Autodesk Inventor part; units mm, degrees
(part 2 of 5)
  line L380 (98.7844, -25.841) -> (96.8773, -27.7481)
  line L381 (94.3702, -25.841) -> (96.2773, -27.7481)
  line L382 (96.5773, -27.7481) -> (96.8773, -27.7481)
  line L383 (96.5773, -27.7481) -> (96.2773, -27.7481)
  line L384 (94.0773, -25.1339) -> (94.0773, -8.3624)
  line L385 (99.0773, -8.3624) -> (99.0773, -25.1339)
  arc A154 (94.3702, -7.6553) -> (94.0773, -8.3624) centre (95.0773, -8.3624) ccw
  line L386 (94.3702, -7.6553) -> (96.2773, -5.7481)
  line L387 (96.5773, -5.7481) -> (96.2773, -5.7481)
  line L388 (96.5773, -5.7481) -> (96.8773, -5.7481)
  arc A155 (99.0773, -8.3624) -> (98.7844, -7.6553) centre (98.0773, -8.3624) ccw
  line L389 (98.7844, -7.6553) -> (96.8773, -5.7481)
  arc A156 (123.5844, -1.041) -> (123.8773, -0.3339) centre (122.8773, -0.3339) ccw
  arc A157 (118.8773, -0.3339) -> (119.1702, -1.041) centre (119.8773, -0.3339) ccw
  line L390 (123.5844, -1.041) -> (121.6773, -2.9481)
  line L391 (119.1702, -1.041) -> (121.0773, -2.9481)
  line L392 (121.3773, -2.9481) -> (121.6773, -2.9481)
  line L393 (121.3773, -2.9481) -> (121.0773, -2.9481)
  line L394 (118.8773, -0.3339) -> (118.8773, 16.4376)
  line L395 (123.8773, 16.4376) -> (123.8773, -0.3339)
  arc A158 (119.1702, 17.1447) -> (118.8773, 16.4376) centre (119.8773, 16.4376) ccw
  line L396 (119.1702, 17.1447) -> (121.0773, 19.0519)
  line L397 (121.3773, 19.0519) -> (121.0773, 19.0519)
  line L398 (121.3773, 19.0519) -> (121.6773, 19.0519)
  arc A159 (123.8773, 16.4376) -> (123.5844, 17.1447) centre (122.8773, 16.4376) ccw
  line L399 (123.5844, 17.1447) -> (121.6773, 19.0519)
  arc A160 (123.5844, -25.841) -> (123.8773, -25.1339) centre (122.8773, -25.1339) ccw
  arc A161 (118.8773, -25.1339) -> (119.1702, -25.841) centre (119.8773, -25.1339) ccw
  line L400 (123.5844, -25.841) -> (121.6773, -27.7481)
  line L401 (119.1702, -25.841) -> (121.0773, -27.7481)
  line L402 (121.3773, -27.7481) -> (121.6773, -27.7481)
  line L403 (121.3773, -27.7481) -> (121.0773, -27.7481)
  line L404 (118.8773, -25.1339) -> (118.8773, -8.3624)
  line L405 (123.8773, -8.3624) -> (123.8773, -25.1339)
  arc A162 (119.1702, -7.6553) -> (118.8773, -8.3624) centre (119.8773, -8.3624) ccw
  line L406 (119.1702, -7.6553) -> (121.0773, -5.7481)
  line L407 (121.3773, -5.7481) -> (121.0773, -5.7481)
  line L408 (121.3773, -5.7481) -> (121.6773, -5.7481)
  arc A163 (123.8773, -8.3624) -> (123.5844, -7.6553) centre (122.8773, -8.3624) ccw
  line L409 (123.5844, -7.6553) -> (121.6773, -5.7481)
  arc A164 (99.8844, -31.3553) -> (100.5916, -31.6481) centre (100.5916, -30.6481) ccw
  arc A165 (100.5916, -26.6481) -> (99.8844, -26.941) centre (100.5916, -27.6481) ccw
  line L410 (99.8844, -31.3553) -> (97.9773, -29.4481)
  line L411 (99.8844, -26.941) -> (97.9773, -28.8481)
  line L412 (97.9773, -29.1481) -> (97.9773, -29.4481)
  line L413 (97.9773, -29.1481) -> (97.9773, -28.8481)
  line L414 (100.5916, -26.6481) -> (117.3631, -26.6481)
  line L415 (117.3631, -31.6481) -> (100.5916, -31.6481)
  arc A166 (118.0702, -26.941) -> (117.3631, -26.6481) centre (117.3631, -27.6481) ccw
  line L416 (118.0702, -26.941) -> (119.9773, -28.8481)
  line L417 (119.9773, -29.1481) -> (119.9773, -28.8481)
  line L418 (119.9773, -29.1481) -> (119.9773, -29.4481)
  arc A167 (117.3631, -31.6481) -> (118.0702, -31.3553) centre (117.3631, -30.6481) ccw
  line L419 (118.0702, -31.3553) -> (119.9773, -29.4481)
  line L420 (-36.3227, 6.9519) -> (-35.3227, 6.9519)
  line L421 (-35.3227, 6.9519) -> (-33.3227, 4.9519)
  line L422 (-33.3227, 4.9519) -> (-33.3227, 3.9519)
  line L423 (-33.3227, 3.9519) -> (-35.3227, 1.9519)
  line L424 (-35.3227, 1.9519) -> (-36.3227, 1.9519)
  line L425 (-36.3227, 1.9519) -> (-38.3227, 3.9519)
  line L426 (-38.3227, 3.9519) -> (-38.3227, 4.9519)
  line L427 (-38.3227, 4.9519) -> (-36.3227, 6.9519)
  line L428 (-36.3227, -13.0481) -> (-35.3227, -13.0481)
  line L429 (-35.3227, -13.0481) -> (-33.3227, -15.0481)
  line L430 (-33.3227, -15.0481) -> (-33.3227, -16.0481)
  line L431 (-33.3227, -16.0481) -> (-35.3227, -18.0481)
  line L432 (-35.3227, -18.0481) -> (-36.3227, -18.0481)
  line L433 (-36.3227, -18.0481) -> (-38.3227, -16.0481)
  line L434 (-38.3227, -16.0481) -> (-38.3227, -15.0481)
  line L435 (-38.3227, -15.0481) -> (-36.3227, -13.0481)
  line L436 (47.7773, 6.9519) -> (48.7773, 6.9519)
  line L437 (48.7773, 6.9519) -> (50.7773, 4.9519)
  line L438 (50.7773, 4.9519) -> (50.7773, 3.9519)
  line L439 (50.7773, 3.9519) -> (48.7773, 1.9519)
  line L440 (48.7773, 1.9519) -> (47.7773, 1.9519)
  line L441 (47.7773, 1.9519) -> (45.7773, 3.9519)
  line L442 (45.7773, 3.9519) -> (45.7773, 4.9519)
  line L443 (45.7773, 4.9519) -> (47.7773, 6.9519)
  line L444 (47.7773, -13.0481) -> (48.7773, -13.0481)
  line L445 (48.7773, -13.0481) -> (50.7773, -15.0481)
  line L446 (50.7773, -15.0481) -> (50.7773, -16.0481)
  line L447 (50.7773, -16.0481) -> (48.7773, -18.0481)
  line L448 (48.7773, -18.0481) -> (47.7773, -18.0481)
  line L449 (47.7773, -18.0481) -> (45.7773, -16.0481)
  line L450 (45.7773, -16.0481) -> (45.7773, -15.0481)
  line L451 (45.7773, -15.0481) -> (47.7773, -13.0481)
  arc A168 (-133.0156, -6.7553) -> (-132.3084, -7.0481) centre (-132.3084, -6.0481) ccw
  arc A169 (-132.3084, -2.0481) -> (-133.0156, -2.341) centre (-132.3084, -3.0481) ccw
  line L452 (-133.0156, -6.7553) -> (-134.9227, -4.8481)
  line L453 (-134.9227, -4.5481) -> (-134.9227, -4.2481)
  line L454 (-134.9227, -4.5481) -> (-134.9227, -4.8481)
  line L455 (-133.0156, -2.341) -> (-134.9227, -4.2481)
  line L456 (-132.3084, -2.0481) -> (-121.5369, -2.0481)
  line L457 (-121.5369, -7.0481) -> (-132.3084, -7.0481)
  arc A170 (-120.8298, -2.341) -> (-121.5369, -2.0481) centre (-121.5369, -3.0481) ccw
  arc A171 (-121.5369, -7.0481) -> (-120.8298, -6.7553) centre (-121.5369, -6.0481) ccw
  line L458 (-120.8298, -6.7553) -> (-118.9227, -4.8481)
  line L459 (-118.9227, -4.5481) -> (-118.9227, -4.8481)
  line L460 (-118.9227, -4.5481) -> (-118.9227, -4.2481)
  line L461 (-120.8298, -2.341) -> (-118.9227, -4.2481)
  arc A172 (-133.7156, -1.641) -> (-133.4227, -0.9339) centre (-134.4227, -0.9339) ccw
  arc A173 (-138.4227, -0.9339) -> (-138.1298, -1.641) centre (-137.4227, -0.9339) ccw
  line L462 (-133.7156, -1.641) -> (-135.6227, -3.5481)
  line L463 (-135.9227, -3.5481) -> (-136.2227, -3.5481)
  line L464 (-135.9227, -3.5481) -> (-135.6227, -3.5481)
  line L465 (-138.1298, -1.641) -> (-136.2227, -3.5481)
  line L466 (-138.4227, -0.9339) -> (-138.4227, 9.8376)
  line L467 (-133.4227, 9.8376) -> (-133.4227, -0.9339)
  arc A174 (-138.1298, 10.5447) -> (-138.4227, 9.8376) centre (-137.4227, 9.8376) ccw
  arc A175 (-133.4227, 9.8376) -> (-133.7156, 10.5447) centre (-134.4227, 9.8376) ccw
  line L468 (-133.7156, 10.5447) -> (-135.6227, 12.4519)
  line L469 (-135.9227, 12.4519) -> (-135.6227, 12.4519)
  line L470 (-135.9227, 12.4519) -> (-136.2227, 12.4519)
  line L471 (-138.1298, 10.5447) -> (-136.2227, 12.4519)
  arc A176 (-151.0156, -6.7553) -> (-150.3084, -7.0481) centre (-150.3084, -6.0481) ccw
  arc A177 (-150.3084, -2.0481) -> (-151.0156, -2.341) centre (-150.3084, -3.0481) ccw
  line L472 (-151.0156, -6.7553) -> (-152.9227, -4.8481)
  line L473 (-152.9227, -4.5481) -> (-152.9227, -4.2481)
  line L474 (-152.9227, -4.5481) -> (-152.9227, -4.8481)
  line L475 (-151.0156, -2.341) -> (-152.9227, -4.2481)
  line L476 (-150.3084, -2.0481) -> (-139.5369, -2.0481)
  line L477 (-139.5369, -7.0481) -> (-150.3084, -7.0481)
  arc A178 (-138.8298, -2.341) -> (-139.5369, -2.0481) centre (-139.5369, -3.0481) ccw
  arc A179 (-139.5369, -7.0481) -> (-138.8298, -6.7553) centre (-139.5369, -6.0481) ccw
  line L478 (-138.8298, -6.7553) -> (-136.9227, -4.8481)
  line L479 (-136.9227, -4.5481) -> (-136.9227, -4.8481)
  line L480 (-136.9227, -4.5481) -> (-136.9227, -4.2481)
  line L481 (-138.8298, -2.341) -> (-136.9227, -4.2481)
  arc A180 (-133.7156, -19.641) -> (-133.4227, -18.9339) centre (-134.4227, -18.9339) ccw
  arc A181 (-138.4227, -18.9339) -> (-138.1298, -19.641) centre (-137.4227, -18.9339) ccw
  line L482 (-133.7156, -19.641) -> (-135.6227, -21.5481)
  line L483 (-135.9227, -21.5481) -> (-136.2227, -21.5481)
  line L484 (-135.9227, -21.5481) -> (-135.6227, -21.5481)
  line L485 (-138.1298, -19.641) -> (-136.2227, -21.5481)
  line L486 (-138.4227, -18.9339) -> (-138.4227, -8.1624)
  line L487 (-133.4227, -8.1624) -> (-133.4227, -18.9339)
  arc A182 (-138.1298, -7.4553) -> (-138.4227, -8.1624) centre (-137.4227, -8.1624) ccw
  arc A183 (-133.4227, -8.1624) -> (-133.7156, -7.4553) centre (-134.4227, -8.1624) ccw
  line L488 (-133.7156, -7.4553) -> (-135.6227, -5.5481)
  line L489 (-135.9227, -5.5481) -> (-135.6227, -5.5481)
  line L490 (-135.9227, -5.5481) -> (-136.2227, -5.5481)
  line L491 (-138.1298, -7.4553) -> (-136.2227, -5.5481)
  arc A184 (-162.5156, 9.2447) -> (-161.8084, 8.9519) centre (-161.8084, 9.9519) ccw
  arc A185 (-161.8084, 13.9519) -> (-162.5156, 13.659) centre (-161.8084, 12.9519) ccw
  line L492 (-162.5156, 9.2447) -> (-164.4227, 11.1519)
  line L493 (-164.4227, 11.4519) -> (-164.4227, 11.7519)
  line L494 (-164.4227, 11.4519) -> (-164.4227, 11.1519)
  line L495 (-162.5156, 13.659) -> (-164.4227, 11.7519)
  line L496 (-161.8084, 13.9519) -> (-151.0369, 13.9519)
  line L497 (-151.0369, 8.9519) -> (-161.8084, 8.9519)
  arc A186 (-150.3298, 13.659) -> (-151.0369, 13.9519) centre (-151.0369, 12.9519) ccw
  arc A187 (-151.0369, 8.9519) -> (-150.3298, 9.2447) centre (-151.0369, 9.9519) ccw
  line L498 (-150.3298, 9.2447) -> (-148.4227, 11.1519)
  line L499 (-148.4227, 11.4519) -> (-148.4227, 11.1519)
  line L500 (-148.4227, 11.4519) -> (-148.4227, 11.7519)
  line L501 (-150.3298, 13.659) -> (-148.4227, 11.7519)
  arc A188 (-179.5156, 9.2447) -> (-178.8084, 8.9519) centre (-178.8084, 9.9519) ccw
  arc A189 (-178.8084, 13.9519) -> (-179.5156, 13.659) centre (-178.8084, 12.9519) ccw
  line L502 (-179.5156, 9.2447) -> (-181.4227, 11.1519)
  line L503 (-181.4227, 11.4519) -> (-181.4227, 11.7519)
  line L504 (-181.4227, 11.4519) -> (-181.4227, 11.1519)
  line L505 (-179.5156, 13.659) -> (-181.4227, 11.7519)
  line L506 (-178.8084, 13.9519) -> (-168.0369, 13.9519)
  line L507 (-168.0369, 8.9519) -> (-178.8084, 8.9519)
  arc A190 (-167.3298, 13.659) -> (-168.0369, 13.9519) centre (-168.0369, 12.9519) ccw
  arc A191 (-168.0369, 8.9519) -> (-167.3298, 9.2447) centre (-168.0369, 9.9519) ccw
  line L508 (-167.3298, 9.2447) -> (-165.4227, 11.1519)
  line L509 (-165.4227, 11.4519) -> (-165.4227, 11.1519)
  line L510 (-165.4227, 11.4519) -> (-165.4227, 11.7519)
  line L511 (-167.3298, 13.659) -> (-165.4227, 11.7519)
  arc A192 (-162.7156, -4.1553) -> (-162.4227, -3.4481) centre (-163.4227, -3.4481) ccw
  arc A193 (-167.4227, -3.4481) -> (-167.1298, -4.1553) centre (-166.4227, -3.4481) ccw
  line L512 (-162.7156, -4.1553) -> (-164.6227, -6.0624)
  line L513 (-164.9227, -6.0624) -> (-165.2227, -6.0624)
  line L514 (-164.9227, -6.0624) -> (-164.6227, -6.0624)
  line L515 (-167.1298, -4.1553) -> (-165.2227, -6.0624)
  line L516 (-167.4227, -3.4481) -> (-167.4227, 7.3234)
  line L517 (-162.4227, 7.3234) -> (-162.4227, -3.4481)
  arc A194 (-167.1298, 8.0305) -> (-167.4227, 7.3234) centre (-166.4227, 7.3234) ccw
  arc A195 (-162.4227, 7.3234) -> (-162.7156, 8.0305) centre (-163.4227, 7.3234) ccw
  line L518 (-162.7156, 8.0305) -> (-164.6227, 9.9376)
  line L519 (-164.9227, 9.9376) -> (-164.6227, 9.9376)
  line L520 (-164.9227, 9.9376) -> (-165.2227, 9.9376)
  line L521 (-167.1298, 8.0305) -> (-165.2227, 9.9376)
  arc A196 (-162.7156, -21.1553) -> (-162.4227, -20.4481) centre (-163.4227, -20.4481) ccw
  arc A197 (-167.4227, -20.4481) -> (-167.1298, -21.1553) centre (-166.4227, -20.4481) ccw
  line L522 (-162.7156, -21.1553) -> (-164.6227, -23.0624)
  line L523 (-164.9227, -23.0624) -> (-165.2227, -23.0624)
  line L524 (-164.9227, -23.0624) -> (-164.6227, -23.0624)
  line L525 (-167.1298, -21.1553) -> (-165.2227, -23.0624)
  line L526 (-167.4227, -20.4481) -> (-167.4227, -9.6766)
  line L527 (-162.4227, -9.6766) -> (-162.4227, -20.4481)
  arc A198 (-167.1298, -8.9695) -> (-167.4227, -9.6766) centre (-166.4227, -9.6766) ccw
  arc A199 (-162.4227, -9.6766) -> (-162.7156, -8.9695) centre (-163.4227, -9.6766) ccw
  line L528 (-162.7156, -8.9695) -> (-164.6227, -7.0624)
  line L529 (-164.9227, -7.0624) -> (-164.6227, -7.0624)
  line L530 (-164.9227, -7.0624) -> (-165.2227, -7.0624)
  line L531 (-167.1298, -8.9695) -> (-165.2227, -7.0624)
  point P0 (-22.4267, -1.12)
  dimension "d362" = 7.5
  dimension "d363" = 17
  dimension "d364" = 7.5
  dimension "d366" = 7.5
  dimension "d367" = 0
  dimension "d368" = 0
  dimension "d369" = 0
  dimension "d370" = 0
  dimension "d371" = 0
  dimension "d372" = 15
  dimension "d373" = 0
  dimension "d374" = 16
  dimension "d375" = 6
  dimension "d376" = 6
  dimension "d377" = 13.6
  dimension "d378" = 16
  dimension "d379" = 6
  dimension "d380" = 15
  dimension "d381" = 0
  dimension "d509" = 22
  dimension "d510" = 25
  dimension "d511" = 24.6
  dimension "d514" = 1
  dimension "d515" = 1
sketch "Clock Front Face Outline" plane through (0, 0, 0) normal (0, 0, 1) x (1, 0, 0)
  line L0 (-365.1075, -11.3808) -> (-85.1075, -11.3808)
  line L1 (-60.1075, -36.3808) -> (-60.1075, -56.3808)
  line L2 (-85.1075, -81.3808) -> (-365.1075, -81.3808)
  line L3 (-390.1075, -56.3808) -> (-390.1075, -36.3808)
  arc A0 (-365.1075, -11.3808) -> (-390.1075, -36.3808) centre (-365.1075, -36.3808) ccw
  arc A1 (-60.1075, -36.3808) -> (-85.1075, -11.3808) centre (-85.1075, -36.3808) ccw
  arc A2 (-85.1075, -81.3808) -> (-60.1075, -56.3808) centre (-85.1075, -56.3808) ccw
  arc A3 (-390.1075, -56.3808) -> (-365.1075, -81.3808) centre (-365.1075, -56.3808) ccw
  point P0 (0, -2.2581)
  dimension "d429" = 330
  dimension "d430" = 70
  dimension "d431" = 25
  measures "d429" distance between parallel lines of L1 L3
  measures "d430" distance between parallel lines of L2 L0
  measures "d431" radius of A0
sketch "Small Segmemt" plane through (0, 0, 0) normal (0, 0, 1) x (1, 0, 0)
  arc A0 (-247.3536, -9.433) -> (-246.6465, -9.7259) centre (-246.6465, -8.7259) ccw
  arc A1 (-246.6465, -4.7259) -> (-247.3536, -5.0187) centre (-246.6465, -5.7259) ccw
  line L0 (-247.3536, -9.433) -> (-249.2607, -7.5259)
  line L1 (-249.2607, -7.2259) -> (-249.2607, -6.9259)
  line L2 (-249.2607, -7.2259) -> (-249.2607, -7.5259)
  line L3 (-247.3536, -5.0187) -> (-249.2607, -6.9259)
  line L4 (-246.6465, -4.7259) -> (-235.875, -4.7259)
  line L5 (-235.875, -9.7259) -> (-246.6465, -9.7259)
  arc A2 (-235.1679, -5.0187) -> (-235.875, -4.7259) centre (-235.875, -5.7259) ccw
  arc A3 (-235.875, -9.7259) -> (-235.1679, -9.433) centre (-235.875, -8.7259) ccw
  line L6 (-235.1679, -9.433) -> (-233.2607, -7.5259)
  line L7 (-233.2607, -7.2259) -> (-233.2607, -7.5259)
  line L8 (-233.2607, -7.2259) -> (-233.2607, -6.9259)
  line L9 (-235.1679, -5.0187) -> (-233.2607, -6.9259)
  point P0 (-225.4266, -6.7349)
  point P1 (-247.0607, -4.7259)
  point P2 (-247.0607, -9.7259)
  point P3 (-235.4607, -4.7259)
  point P4 (-235.4607, -9.7259)
  dimension "d462" = 2.2
  dimension "d463" = 2.2
  dimension "d464" = 2.2
  dimension "d465" = 2.2
  dimension "d466" = 2.2
  dimension "d467" = 2.2
  dimension "d468" = 2.2
  dimension "d469" = 1
  dimension "d470" = 5
  dimension "d471" = 2.2
  dimension "d472" = 2.2
  dimension "d473" = 135
  dimension "d474" = 16
  dimension "d475" = 135
  dimension "d476" = 2.5
  dimension "d477" = 5
  dimension "d478" = 16
  dimension "d479" = 2.2
  dimension "d480" = 0.3
  dimension "d481" = 0.3
  dimension "d482" = 0.3
  dimension "d483" = 0.3
  measures "d462" horizontal distance of point (-247.061, -9.726) L0.end
  measures "d463" horizontal distance of L8.end point (-235.461, -4.726)
  measures "d464" horizontal distance of point (-247.061, -4.726) L1.end
  measures "d465" horizontal distance of L6.end point (-235.461, -9.726)
  measures "d466" horizontal distance of L6.end point (-235.461, -9.726)
  measures "d467" horizontal distance of point (-247.061, -4.726) L1.end
  measures "d468" horizontal distance of point (-247.061, -9.726) L0.end
  measures "d469" radius of A1
  measures "d470" distance of point (-235.461, -9.726) point (-235.461, -4.726)
  measures "d471" horizontal distance of L8.end point (-235.461, -4.726)
  measures "d472" horizontal distance of point (-235.461, -9.726) L7.start
  measures "d473" angle of L5 L6
  measures "d474" horizontal distance of L6.end L1.start
  measures "d475" angle of L4 L9
  measures "d476" vertical distance of L7.start point (-235.461, -9.726)
  measures "d477" distance between parallel lines of L5 L4
  measures "d478" distance of L1.start L7.start
  measures "d479" horizontal distance of point (-247.061, -4.726) L1.start
  measures "d480" distance of L7.start L8.end
  measures "d481" distance of L6.end L7.start
  measures "d482" distance of L1.end L1.start
  measures "d483" distance of L0.end L1.start
sketch "7SegmentOutline" plane through (0, 0, 0) normal (0, 0, 1) x (1, 0, 0)
  line L0 (61.3689, -70.3118) -> (59.4618, -72.219)
  line L1 (80.6547, -69.2118) -> (82.5618, -71.119)
  line L2 (81.4618, -72.219) -> (79.5547, -70.3118)
  line L3 (79.5547, -74.7261) -> (81.4618, -72.819)
  line L4 (81.4618, -72.819) -> (81.4618, -72.219)
  line L5 (81.4618, -72.219) -> (79.2618, -70.019)
  line L6 (79.5547, -95.1118) -> (81.4618, -97.019)
  line L7 (80.6547, -94.0118) -> (82.5618, -95.919)
  line L8 (60.2689, -94.0118) -> (58.3618, -95.919)
  line L9 (61.3689, -95.1118) -> (59.4618, -97.019)
  line L10 (81.4618, -48.019) -> (81.4618, -47.419)
  line L11 (61.3689, -45.5118) -> (59.4618, -47.419)
  line L12 (59.4618, -47.419) -> (59.4618, -48.019)
  line L13 (59.4618, -48.019) -> (59.4618, -47.419)
  line L14 (61.3689, -49.9261) -> (59.4618, -48.019)
  line L15 (60.2689, -51.0261) -> (58.3618, -49.119)
  line L16 (57.7618, -49.119) -> (55.8547, -51.0261)
  line L17 (55.8547, -69.2118) -> (57.7618, -71.119)
  line L18 (57.7618, -71.119) -> (58.3618, -71.119)
  line L19 (58.3618, -71.119) -> (60.2689, -69.2118)
  line L20 (60.2689, -75.8261) -> (58.3618, -73.919)
  line L21 (57.7618, -73.919) -> (55.8547, -75.8261)
  line L22 (55.5618, -76.5332) -> (55.5618, -93.3047)
  line L23 (55.8547, -94.0118) -> (57.7618, -95.919)
  line L24 (59.4618, -97.019) -> (59.4618, -97.619)
  line L25 (59.4618, -97.619) -> (61.3689, -99.5261)
  line L26 (62.076, -99.819) -> (78.8476, -99.819)
  line L27 (79.5547, -99.5261) -> (81.4618, -97.619)
  line L28 (81.4618, -97.619) -> (81.4618, -97.019)
  line L29 (82.5618, -95.919) -> (83.1618, -95.919)
  line L30 (83.1618, -95.919) -> (85.0689, -94.0118)
  line L31 (85.3618, -93.3047) -> (85.3618, -76.5332)
  line L32 (85.0689, -75.8261) -> (83.1618, -73.919)
  line L33 (83.1618, -73.919) -> (82.5618, -73.919)
  line L34 (82.5618, -73.919) -> (80.6547, -75.8261)
  line L35 (81.4618, -72.819) -> (81.4618, -72.219)
  line L36 (83.1618, -71.119) -> (85.0689, -69.2118)
  line L37 (85.3618, -68.5047) -> (85.3618, -51.7332)
  line L38 (85.0689, -51.0261) -> (83.1618, -49.119)
  line L39 (83.1618, -49.119) -> (82.5618, -49.119)
  line L40 (82.5618, -49.119) -> (80.6547, -51.0261)
  line L41 (81.4618, -48.019) -> (81.4618, -47.419)
  line L42 (62.076, -45.219) -> (78.8476, -45.219)
  line L43 (55.5618, -51.7332) -> (55.5618, -68.5047)
  line L44 (81.4618, -47.419) -> (79.5547, -45.5118)
  line L45 (81.4618, -48.019) -> (79.5547, -49.9261)
  line L46 (82.5618, -71.119) -> (83.1618, -71.119)
  arc A0 (55.8547, -51.0261) -> (55.5618, -51.7332) centre (56.5618, -51.7332) ccw
  arc A1 (62.076, -45.219) -> (61.3689, -45.5118) centre (62.076, -46.219) ccw
  arc A2 (79.5547, -45.5118) -> (78.8476, -45.219) centre (78.8476, -46.219) ccw
  arc A3 (85.3618, -51.7332) -> (85.0689, -51.0261) centre (84.3618, -51.7332) ccw
  arc A4 (85.0689, -69.2118) -> (85.3618, -68.5047) centre (84.3618, -68.5047) ccw
  arc A5 (85.3618, -76.5332) -> (85.0689, -75.8261) centre (84.3618, -76.5332) ccw
  arc A6 (85.0689, -94.0118) -> (85.3618, -93.3047) centre (84.3618, -93.3047) ccw
  arc A7 (78.8476, -99.819) -> (79.5547, -99.5261) centre (78.8476, -98.819) ccw
  arc A8 (61.3689, -99.5261) -> (62.076, -99.819) centre (62.076, -98.819) ccw
  arc A9 (55.5618, -93.3047) -> (55.8547, -94.0118) centre (56.5618, -93.3047) ccw
  arc A10 (55.8547, -75.8261) -> (55.5618, -76.5332) centre (56.5618, -76.5332) ccw
  arc A11 (55.5618, -68.5047) -> (55.8547, -69.2118) centre (56.5618, -68.5047) ccw
  line L47 (57.7618, -49.119) -> (58.3618, -49.119)
  line L48 (59.4618, -72.219) -> (59.4618, -72.819)
  line L49 (61.3689, -74.7261) -> (59.4618, -72.819)
  line L50 (57.7618, -73.919) -> (58.3618, -73.919)
  line L51 (57.7618, -95.919) -> (58.3618, -95.919)
  line L52 (62.6618, -51.319) -> (78.2618, -51.319)
  line L53 (80.3618, -51.7332) -> (80.3618, -68.5047)
  line L54 (78.2618, -68.919) -> (62.6618, -68.919)
  line L55 (60.5618, -68.5047) -> (60.5618, -51.7332)
  line L56 (62.076, -50.219) -> (78.8476, -50.219)
  line L57 (79.2618, -52.319) -> (79.2618, -67.919)
  line L58 (78.8476, -70.019) -> (62.076, -70.019)
  line L59 (61.6618, -67.919) -> (61.6618, -52.319)
  line L60 (62.6618, -76.119) -> (78.2618, -76.119)
  line L61 (80.3618, -76.5332) -> (80.3618, -93.3047)
  line L62 (78.2618, -93.719) -> (62.6618, -93.719)
  line L63 (60.5618, -93.3047) -> (60.5618, -76.5332)
  line L64 (62.076, -94.819) -> (78.8476, -94.819)
  line L65 (79.2618, -92.719) -> (79.2618, -77.119)
  line L66 (78.8476, -75.019) -> (62.076, -75.019)
  line L67 (61.6618, -77.119) -> (61.6618, -92.719)
  arc A12 (80.6547, -51.0261) -> (80.3618, -51.7332) centre (81.3618, -51.7332) ccw
  arc A13 (78.8476, -50.219) -> (79.5547, -49.9261) centre (78.8476, -49.219) ccw
  arc A14 (61.3689, -49.9261) -> (62.076, -50.219) centre (62.076, -49.219) ccw
  arc A15 (60.5618, -51.7332) -> (60.2689, -51.0261) centre (59.5618, -51.7332) ccw
  arc A16 (80.3618, -68.5047) -> (80.6547, -69.2118) centre (81.3618, -68.5047) ccw
  arc A17 (80.6547, -75.8261) -> (80.3618, -76.5332) centre (81.3618, -76.5332) ccw
  arc A18 (79.5547, -70.3118) -> (78.8476, -70.019) centre (78.8476, -71.019) ccw
  arc A19 (78.8476, -75.019) -> (79.5547, -74.7261) centre (78.8476, -74.019) ccw
  arc A20 (61.3689, -74.7261) -> (62.076, -75.019) centre (62.076, -74.019) ccw
  arc A21 (62.076, -70.019) -> (61.3689, -70.3118) centre (62.076, -71.019) ccw
  arc A22 (60.5618, -76.5332) -> (60.2689, -75.8261) centre (59.5618, -76.5332) ccw
  arc A23 (60.2689, -69.2118) -> (60.5618, -68.5047) centre (59.5618, -68.5047) ccw
  arc A24 (62.6618, -76.119) -> (61.6618, -77.119) centre (62.6618, -77.119) ccw
  arc A25 (79.2618, -77.119) -> (78.2618, -76.119) centre (78.2618, -77.119) ccw
  arc A26 (78.2618, -93.719) -> (79.2618, -92.719) centre (78.2618, -92.719) ccw
  arc A27 (79.5547, -95.1118) -> (78.8476, -94.819) centre (78.8476, -95.819) ccw
  arc A28 (61.6618, -92.719) -> (62.6618, -93.719) centre (62.6618, -92.719) ccw
  arc A29 (60.2689, -94.0118) -> (60.5618, -93.3047) centre (59.5618, -93.3047) ccw
  arc A30 (62.076, -94.819) -> (61.3689, -95.1118) centre (62.076, -95.819) ccw
  arc A31 (79.2618, -52.319) -> (78.2618, -51.319) centre (78.2618, -52.319) ccw
  arc A32 (62.6618, -51.319) -> (61.6618, -52.319) centre (62.6618, -52.319) ccw
  arc A33 (78.2618, -68.919) -> (79.2618, -67.919) centre (78.2618, -67.919) ccw
  arc A34 (61.6618, -67.919) -> (62.6618, -68.919) centre (62.6618, -67.919) ccw
  arc A35 (80.3618, -93.3047) -> (80.6547, -94.0118) centre (81.3618, -93.3047) ccw
  point P0 (-253.3255, -154.094)
  point P1 (80.3618, -51.319)
  point P2 (61.6618, -50.219)
  point P3 (60.5618, -51.319)
  point P4 (79.2618, -50.219)
  point P5 (60.5618, -68.919)
  point P6 (61.6618, -70.019)
  point P7 (61.6618, -75.019)
  point P8 (60.5618, -76.119)
  point P9 (60.5618, -93.719)
  point P10 (61.6618, -94.819)
  point P11 (79.2618, -94.819)
  point P12 (80.3618, -93.719)
  point P13 (80.3618, -68.919)
  point P14 (80.3618, -76.119)
  point P15 (61.6618, -75.019)
  dimension "d139" = 1.1
  dimension "d1139" = 1.5556
  dimension "d1140" = 1.5556
  dimension "d1143" = 1.5556
  dimension "d1144" = 1.5556
  dimension "d1145" = 90
  dimension "d1198" = 135
  dimension "d1199" = 1.5556
  dimension "d1210" = 90
  dimension "d1216" = 90
  dimension "d1233" = 90
  dimension "d1259" = 135
  dimension "d1260" = 135
  dimension "d1135" = 29.8
  dimension "d1136" = 29.8
  dimension "d1137" = 54.6
  dimension "d1146" = 2.2
  dimension "d1147" = 0.6
  dimension "d1150" = 0.6
  dimension "d1153" = 0.6
  dimension "d1154" = 2.2
  dimension "d1155" = 25.9
  dimension "d1156" = 25.9
  dimension "d1157" = 2.2
  dimension "d1158" = 0.6
  dimension "d1159" = 2.2
  dimension "d1160" = 2.2
  dimension "d1161" = 0.6
  dimension "d1162" = 2.2
  dimension "d1163" = 2.2
  dimension "d1164" = 0.6
  dimension "d1165" = 2.2
  dimension "d1166" = 2.2
  dimension "d1167" = 0.6
  dimension "d1168" = 2.2
  dimension "d1169" = 2.2
  dimension "d1170" = 2.2
  dimension "d1171" = 2.2
  dimension "d1172" = 2.2
  dimension "d1173" = 2.2
  dimension "d1175" = 2.8
  dimension "d1176" = 22
  dimension "d1177" = 22
  dimension "d1178" = 25.9
  dimension "d1179" = 2.2
  dimension "d1180" = 0.6
  dimension "d1181" = 2.2
  dimension "d1182" = 2.2
  dimension "d1183" = 0.6
  dimension "d1184" = 2.2
  dimension "d1188" = 2.2
  dimension "d1189" = 0.6
  dimension "d1190" = 2.2
  dimension "d1193" = 2.2
  dimension "d1194" = 0.6
  dimension "d1195" = 0
  dimension "d1196" = 0
  dimension "d1200" = 2.2
  dimension "d1201" = 0
  dimension "d1202" = 0
  dimension "d1205" = 0
  dimension "d1206" = 0
  dimension "d1207" = 0
  dimension "d1208" = 135
  dimension "d1209" = 90
  dimension "d1211" = 2.2
  dimension "d1212" = 0.6
  dimension "d1213" = 16.7716
  dimension "d1214" = 16.7716
  dimension "d1215" = 16.7716
  dimension "d1217" = 135
  dimension "d1218" = 16.7716
  dimension "d1219" = 1
  dimension "d1221" = 135
  dimension "d1222" = 1
  dimension "d1223" = 2.2
  dimension "d1224" = 2.2
  measures "d1135" distance between parallel lines of L31 L22
  measures "d1136" distance between parallel lines of L37 L43
  measures "d1137" distance between parallel lines of L42 L26
  measures "d1146" distance from line of L33.start L31
  measures "d1147" distance of L33.start L33.end
  measures "d1150" distance of L4.start L4.end
  measures "d1153" distance of L46.start L46.end
  measures "d1154" distance from line of L37 L46.end
  measures "d1155" distance between parallel lines of L42 L46
  measures "d1156" distance between parallel lines of L42 L18
  measures "d1157" distance from line of L42 L10.end
  measures "d1158" distance of L10.start L10.end
  measures "d1159" horizontal distance of L10.start point (79.262, -50.219)
  measures "d1160" horizontal distance of point (80.362, -51.319) L39.end
  measures "d1161" distance of L39.start L39.end
  measures "d1162" distance from line of L37 L39.start
  measures "d1163" horizontal distance of L29.start point (80.362, -93.719)
  measures "d1164" distance of L29.start L29.end
  measures "d1165" distance from line of L31 L29.end
  measures "d1166" horizontal distance of L28.end point (79.262, -94.819)
  measures "d1167" distance of L27.end L28.end
  measures "d1168" distance from line of L26 L27.end
  measures "d1169" horizontal distance of L28.end point (79.262, -94.819)
  measures "d1170" horizontal distance of L29.start point (80.362, -93.719)
  measures "d1171" horizontal distance of L33.end point (80.362, -76.119)
  measures "d1172" horizontal distance of point (80.362, -68.919) L46.start
  measures "d1173" horizontal distance of L4.end L5.end
  measures "d1175" distance between parallel lines of L46 L33
  measures "d1176" distance from line of L29.start L33
  measures "d1177" distance between parallel lines of L39 L46
  measures "d1178" distance from line of L26 L33.end
  measures "d1179" distance from line of L42 L12.start
  measures "d1180" distance of L12.start L12.end
  measures "d1181" horizontal distance of point (61.662, -50.219) L12.end
  measures "d1182" horizontal distance of point (60.562, -51.319) point (58.362, -49.119)
  measures "d1183" distance of point (57.762, -49.119) point (58.362, -49.119)
  measures "d1184" distance from line of L43 point (57.762, -49.119)
  measures "d1188" distance from line of L17.end L43
  measures "d1189" distance of L17.end L18.end
  measures "d1190" horizontal distance of L18.end point (60.562, -68.919)
  measures "d1193" horizontal distance of point (61.662, -70.019) point (59.462, -72.219)
  measures "d1194" distance of point (59.462, -72.219) point (59.462, -72.819)
  measures "d1195" distance of point (59.462, -72.219) point (59.462, -72.219)
  measures "d1196" distance of point (59.462, -72.819) point (59.462, -72.819)
  measures "d1200" horizontal distance of point (58.362, -73.919) point (60.562, -76.119)
  measures "d1201" distance of point (61.662, -75.019) point (61.662, -75.019)
  measures "d1202" distance of point (61.662, -75.019) point (61.662, -75.019)
  measures "d1205" distance of point (58.362, -73.919) point (58.362, -73.919)
  measures "d1206" distance of point (57.762, -73.919) point (57.762, -73.919)
  measures "d1207" distance of point (58.362, -73.919) point (58.362, -73.919)
  measures "d1208" angle of L17 L43
  measures "d1211" distance from line of point (57.762, -73.919) L22
  measures "d1212" distance of point (57.762, -73.919) point (58.362, -73.919)
  measures "d1213" distance of L43.start L43.end
  measures "d1214" distance of L37.start L37.end
  measures "d1215" distance of L31.start L31.end
  measures "d1218" distance of L22.start L22.end
  measures "d1219" radius of A10
  measures "d1222" radius of A9
  measures "d1223" distance from line of point (57.762, -95.919) L22
  measures "d1224" horizontal distance of point (60.562, -93.719) point (58.362, -95.919)
sketch "Cable Trench" plane through (0, 0, 0) normal (0, 0, 1) x (1, 0, 0)
  line L0 (44.8, -0.8) -> (44.8, 0.2)
  line L1 (49.9831, -0.8) -> (44.8, -0.8)
  line L2 (44.8, 0.2) -> (50.3, 0.2)
  line L3 (50.8, 1.7) -> (50.8, 0.7)
  arc A0 (50.3, 0.2) -> (50.8, 0.7) centre (50.3, 0.7) ccw
  line L4 (49.9831, -0.8) -> (51.3, -0.8)
  line L5 (52.3, 1.2) -> (52.3, 1.2)
  arc A1 (52.3, 1.2) -> (51.8, 0.7) centre (52.3, 0.7) ccw
  arc A2 (51.3, -0.8) -> (51.8, -0.3) centre (51.3, -0.3) ccw
  arc A3 (52.8, 0.7) -> (52.3, 1.2) centre (52.3, 0.7) ccw
  line L6 (53.063, 2.2) -> (51.3, 2.2)
  line L7 (53.063, 2.2) -> (53.3, 2.2)
  arc A4 (53.8, 1.7) -> (53.3, 2.2) centre (53.3, 1.7) ccw
  line L8 (53.8, 1.7) -> (53.8, -1.3)
  line L9 (55.1, -2.8) -> (55.3, -2.8)
  line L10 (55.1, -2.8) -> (54.063, -2.8)
  line L11 (61.7623, 0.2) -> (61.7623, -0.8)
  line L12 (56.1, 0.2) -> (61.7623, 0.2)
  line L13 (61.7623, -0.8) -> (56.3, -0.8)
  line L14 (56.1, 0.2) -> (57.1, 0.2)
  line L15 (56.1, 0.2) -> (55.3, 0.2)
  line L16 (54.3, -1.8) -> (54.3, -1.8)
  arc A5 (55.3, -2.8) -> (55.8, -2.3) centre (55.3, -2.3) ccw
  arc A6 (54.3, -1.8) -> (54.8, -1.3) centre (54.3, -1.3) ccw
  line L17 (55.8, -2.3) -> (55.8, -1.3)
  line L18 (54.8, -0.3) -> (54.8, -1.3)
  arc A7 (56.3, -0.8) -> (55.8, -1.3) centre (56.3, -1.3) ccw
  arc A8 (55.3, 0.2) -> (54.8, -0.3) centre (55.3, -0.3) ccw
  arc A9 (53.8, -1.3) -> (54.3, -1.8) centre (54.3, -1.3) ccw
  line L19 (54.063, -2.8) -> (53.3, -2.8)
  arc A10 (52.8, -2.3) -> (53.3, -2.8) centre (53.3, -2.3) ccw
  line L20 (52.8, -2.3) -> (52.8, 0.7)
  line L21 (51.8, -0.3) -> (51.8, 0.7)
  arc A11 (51.3, 2.2) -> (50.8, 1.7) centre (51.3, 1.7) ccw
  point P0 (153.0768, 0)
  dimension "d1507" = 0
  dimension "d1515" = 0
  dimension "d1516" = 0
  dimension "d1517" = 0
  dimension "d1518" = 0
  dimension "d1521" = 5
  dimension "d1508" = 1
  dimension "d1509" = 1
  dimension "d1510" = 1
  dimension "d1511" = 1
  dimension "d1513" = 1
  dimension "d1514" = 1
  dimension "d1519" = 0.5
  dimension "d1520" = 0.5
  dimension "d1522" = 1
  dimension "d1523" = 1
  dimension "d1524" = 1
  dimension "d1525" = 3
  dimension "d1526" = 3
  dimension "d1527" = 1
  dimension "d1529" = 6.9623
  measures "d1508" distance between parallel lines of L21 L3
  measures "d1510" distance between parallel lines of L8 L20
  measures "d1513" distance between parallel lines of L5 L2
  measures "d1519" radius of A0
  measures "d1520" radius of A7
  measures "d1522" distance between parallel lines of L20 L21
  measures "d1523" distance between parallel lines of L18 L8
  measures "d1524" distance between parallel lines of L18 L17
  measures "d1525" horizontal distance of point (54.3, -1.3) A11.centre
  measures "d1526" horizontal distance of A2.centre point (54.3, -1.3)
  measures "d1527" distance of L11.start L11.end
  measures "d1529" distance between parallel lines of L18 L11
sketch "Cable Trench Long" plane through (0, 0, 0) normal (0, 0, 1) x (1, 0, 0)
  line L0 (6.4924, 2.4404) -> (9.9924, 2.4404)
  arc A0 (10.4924, 1.9404) -> (9.9924, 2.4404) centre (9.9924, 1.9404) ccw
  line L1 (11.9924, 7.9404) -> (11.9924, -3.1373)
  line L2 (10.4924, -5.3873) -> (10.4924, 1.9404)
  arc A1 (6.4924, 2.4404) -> (5.9924, 1.9404) centre (6.4924, 1.9404) ccw
  line L3 (5.9924, -0.3096) -> (5.9924, 1.9404)
  line L4 (-2.0076, -0.8096) -> (-2.0076, 0.1904)
  line L5 (-2.0076, 0.1904) -> (3.9924, 0.1904)
  arc A2 (3.9924, 0.1904) -> (4.4924, 0.6904) centre (3.9924, 0.6904) ccw
  line L6 (4.4924, 3.4404) -> (4.4924, 0.6904)
  line L7 (-2.0076, -0.8096) -> (5.4924, -0.8096)
  line L8 (16.4924, -0.3096) -> (16.4924, -3.1373)
  line L9 (24.4924, -0.8096) -> (18.4924, -0.8096)
  line L10 (17.9924, -4.6373) -> (17.9924, -1.3096)
  arc A3 (11.9924, -3.1373) -> (12.4924, -3.6373) centre (12.4924, -3.1373) ccw
  line L11 (12.4924, -3.6373) -> (15.9924, -3.6373)
  line L12 (16.9924, 0.1904) -> (24.4924, 0.1904)
  line L13 (10.4924, 7.9404) -> (10.4924, 4.4404)
  line L14 (11.9924, -5.6373) -> (11.9924, -11.1373)
  line L15 (10.4924, -11.1373) -> (10.4924, -4.6373)
  line L16 (17.4924, -5.1373) -> (12.4924, -5.1373)
  arc A4 (12.4924, -5.1373) -> (11.9924, -5.6373) centre (12.4924, -5.6373) ccw
  line L17 (4.9924, 3.9404) -> (9.9924, 3.9404)
  arc A5 (9.9924, 3.9404) -> (10.4924, 4.4404) centre (9.9924, 4.4404) ccw
  line L18 (10.4924, -11.1373) -> (11.9924, -11.1373)
  line L19 (10.4924, 7.9404) -> (11.9924, 7.9404)
  line L20 (24.4924, -0.8096) -> (24.4924, 0.1904)
  arc A6 (5.4924, -0.8096) -> (5.9924, -0.3096) centre (5.4924, -0.3096) ccw
  arc A7 (4.9924, 3.9404) -> (4.4924, 3.4404) centre (4.9924, 3.4404) ccw
  arc A8 (17.4924, -5.1373) -> (17.9924, -4.6373) centre (17.4924, -4.6373) ccw
  arc A9 (15.9924, -3.6373) -> (16.4924, -3.1373) centre (15.9924, -3.1373) ccw
  arc A10 (16.9924, 0.1904) -> (16.4924, -0.3096) centre (16.9924, -0.3096) ccw
  arc A11 (18.4924, -0.8096) -> (17.9924, -1.3096) centre (18.4924, -1.3096) ccw
  point P0 (153.0768, 0)
  dimension "d1898" = 1
  dimension "d1899" = 1.5
  dimension "d1900" = 1.5
  dimension "d1901" = 1.5
  dimension "d1902" = 1.5
  dimension "d1903" = 1.5
  dimension "d1904" = 1.5
  dimension "d1905" = 1
  dimension "d1906" = 6.5
  dimension "d1907" = 4.5
  dimension "d1908" = 4.5
  dimension "d1909" = 6.5
  dimension "d1910" = 4
  dimension "d1911" = 6
  dimension "d1912" = 6.0777
  dimension "d1913" = 0.5
  dimension "d1914" = 7.75
  dimension "d1915" = 10.3277
  dimension "d1916" = 7.75
  dimension "d1917" = 10.3277
  dimension "d1921" = 0
  measures "d1898" distance between parallel lines of L7 L5
  measures "d1899" distance between parallel lines of L6 L3
  measures "d1900" distance between parallel lines of L0 L17
  measures "d1901" distance between parallel lines of L1 L13
  measures "d1902" distance between parallel lines of L14 L15
  measures "d1903" distance between parallel lines of L16 L11
  measures "d1904" distance between parallel lines of L8 L10
  measures "d1905" distance between parallel lines of L12 L9
  measures "d1906" distance between parallel lines of L6 L4
  measures "d1907" distance between parallel lines of L2 L3
  measures "d1908" distance between parallel lines of L8 L14
  measures "d1909" distance between parallel lines of L20 L10
  measures "d1910" distance between parallel lines of L17 L19
  measures "d1911" distance between parallel lines of L16 L18
  measures "d1912" distance between parallel lines of L11 L0
  measures "d1913" radius of A5
  measures "d1914" distance between parallel lines of L19 L5
  measures "d1915" distance between parallel lines of L18 L7
  measures "d1916" distance between parallel lines of L12 L19
  measures "d1917" distance between parallel lines of L9 L18
  measures "d1921" distance of L9.start L20.start
sketch "CableCutouts" plane through (0, 0, 0) normal (0, 0, 1) x (1, 0, 0)
  line L0 (-137.6, 22) -> (-136.6, 22)
  line L1 (-136.6, 22) -> (-136.6, 20.9)
  line L2 (-136.6, 20.9) -> (-137.6, 20.9)
  line L3 (-137.6, 20.9) -> (-137.6, 22)
  line L4 (-143.3, 7.3) -> (-142.2, 7.3)
  line L5 (-142.2, 7.3) -> (-142.2, 6.3)
  line L6 (-142.2, 6.3) -> (-143.3, 6.3)
  line L7 (-143.3, 6.3) -> (-143.3, 7.3)
  line L8 (-128.6, 3.3) -> (-127.6, 3.3)
  line L9 (-127.6, 3.3) -> (-127.6, 2.2)
  line L10 (-127.6, 2.2) -> (-128.6, 2.2)
  line L11 (-128.6, 2.2) -> (-128.6, 3.3)
  line L12 (-124.6, 14.9) -> (-123.5, 14.9)
  line L13 (-123.5, 14.9) -> (-123.5, 13.9)
  line L14 (-123.5, 13.9) -> (-124.6, 13.9)
  line L15 (-124.6, 13.9) -> (-124.6, 14.9)
  line L16 (-140.6, -2.8) -> (-139.6, -2.8)
  line L17 (-139.6, -2.8) -> (-139.6, -3.9)
  line L18 (-139.6, -3.9) -> (-140.6, -3.9)
  line L19 (-140.6, -3.9) -> (-140.6, -2.8)
  line L20 (-143.3, -17.5) -> (-142.2, -17.5)
  line L21 (-142.2, -17.5) -> (-142.2, -18.5)
  line L22 (-142.2, -18.5) -> (-143.3, -18.5)
  line L23 (-143.3, -18.5) -> (-143.3, -17.5)
  line L24 (-128.6, -21.5) -> (-127.6, -21.5)
  line L25 (-127.6, -21.5) -> (-127.6, -22.6)
  line L26 (-127.6, -22.6) -> (-128.6, -22.6)
  line L27 (-128.6, -22.6) -> (-128.6, -21.5)
  line L28 (-124.6, -9.9) -> (-123.5, -9.9)
  line L29 (-123.5, -9.9) -> (-123.5, -10.9)
  line L30 (-123.5, -10.9) -> (-124.6, -10.9)
  line L31 (-124.6, -10.9) -> (-124.6, -9.9)
  point P0 (153.0768, 0)
  dimension "d1699" = 0.5
  dimension "d1700" = 0.5
  dimension "d1701" = 8.75
  dimension "d1702" = 1
  dimension "d1703" = 1
  dimension "d1704" = 2
  dimension "d1705" = 2
  dimension "d1706" = 2
  dimension "d1707" = 0
  dimension "d1708" = 1
  dimension "d1709" = 1
  dimension "d1710" = 3.7142
  dimension "d1711" = 0
  dimension "d1712" = 1
  dimension "d1713" = 1
  dimension "d1714" = 0.3
  dimension "d1715" = 1
  dimension "d1716" = 1
  dimension "d1717" = 1
  dimension "d1718" = 1
  dimension "d1719" = 3.5
  dimension "d1720" = 3.4261
  dimension "d1721" = 1
  dimension "d1722" = 2
  dimension "d1809" = 1
  dimension "d1810" = 1
  dimension "d1811" = 1
  dimension "d1812" = 1
  dimension "d1814" = 1
  dimension "d1815" = 1
  measures "d1809" distance between parallel lines of L6 L4
  measures "d1810" distance between parallel lines of L14 L12
  measures "d1811" distance between parallel lines of L1 L3
  measures "d1812" distance between parallel lines of L30 L28
  measures "d1814" distance between parallel lines of L22 L20
  measures "d1815" distance between parallel lines of L25 L27
sketch "Sketch1" plane through (0, 0, 0) normal (0, 0, 1) x (1, 0, 0)
  line L0 (-140, 35) -> (140, 35)
  line L1 (165, 10) -> (165, -10)
  line L2 (140, -35) -> (-140, -35)
  line L3 (-165, -10) -> (-165, 10)
  arc A0 (-140, 35) -> (-165, 10) centre (-140, 10) ccw
  arc A1 (165, 10) -> (140, 35) centre (140, 10) ccw
  arc A2 (140, -35) -> (165, -10) centre (140, -10) ccw
  arc A3 (-165, -10) -> (-140, -35) centre (-140, -10) ccw
  point P0 (0, 0)
  dimension "d536" = 35
  dimension "d537" = 165
  dimension "d538" = 165
  dimension "d539" = 35
extrude "Extrusion1" add sketch "Sketch1" along normal blind 5